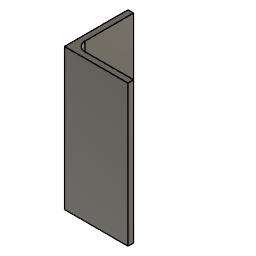
L-45×45×4 (Autodesk Fusion 360 design; units mm, degrees)
Autodesk Fusion 360 part; units mm, degrees
sketch "スケッチ1" plane through (0, 0, 0) normal (0, 0, 1) x (1, 0, 0)
  line L0 (0, 45) -> (0, 0)
  line L1 (4, 10.5) -> (4, 45)
  line L2 (45, 4) -> (10.5, 4)
  line L3 (0, 0) -> (45, 0)
  arc A0 (4, 10.5) -> (10.5, 4) centre (10.5, 10.5) ccw
  line L4 (45, 0) -> (45, 4)
  line L5 (4, 45) -> (0, 45)
extrude "押し出し1" add sketch "スケッチ1" along normal blind 100
